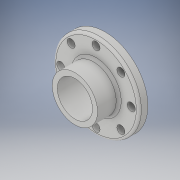
# Autodesk Inventor part: 410571040-T3
Saved by Autodesk Inventor 2017 (Build 210142000, 142)
## iProperties
Part Number: 410571040-T3
Material: 一般
Document SubType Name: Modeling
Designer: user
Density: 1 g/cm^3
Appearance: 預設
Author: user
Autodesk Inventor part; units mm, degrees
ref_plane "YZ Plane" through (0, 0, 0) normal (1, 0, 0) x (0, 1, 0)
ref_plane "XZ Plane" through (0, 0, 0) normal (0, 1, 0) x (-1, 0, 0)
ref_plane "XY Plane" through (0, 0, 0) normal (0, 0, 1) x (1, 0, 0)
sketch "草圖1" plane through (0, 0, 0) normal (1, 0, 0) x (0, 1, 0)
  line L0 (0, 0) -> (45, 0)
  line L1 (45, 0) -> (45, -42)
  line L2 (45, -42) -> (85, -42)
  line L3 (85, -42) -> (85, -60)
  line L4 (85, -60) -> (0, -60)
  line L5 (0, -60) -> (0, 0)
  dimension "d0" = 60
  dimension "d1" = 85
  dimension "d2" = 42
  dimension "d3" = 40
  constraints: 12 end point, 5 perpendicular, 1 horizontal
  measures "d0" distance of L4.end L0.start
  measures "d1" distance of L3.end L4.end
  measures "d2" distance of L0.end L1.end
  measures "d3" distance of L1.end L2.end
revolve "迴轉1" add sketch "草圖1" angle 360 about axis through (0, 0, -60) along (0, 0, 1)
sketch "草圖2" plane through (0, 0, -42) normal (0, 0, 1) x (1, 0, 0)
  circle A0 centre (0, 0) radius 70 construction
  circle A1 centre (0, 70) radius 8
  circle A2 centre (-49.4975, 49.4975) radius 8
  circle A3 centre (-70, 0) radius 8
  circle A4 centre (-49.4975, -49.4975) radius 8
  circle A5 centre (0, -70) radius 8
  circle A6 centre (49.4975, -49.4975) radius 8
  circle A7 centre (70, 0) radius 8
  circle A8 centre (49.4975, 49.4975) radius 8
  dimension "d5" = 140
  dimension "d6" = 16
  dimension "d7" = 70
  dimension "d12" = 360
  constraints: 8 centre point, 6 coincident, 1 vertical alignment, 25 other
  measures "d6" diameter of A1
  measures "d7" distance of A1.centre point (0, 0)
extrude "擠出1" cut sketch "草圖2" against normal up to next
sketch "草圖4" plane through (0, 0, 0) normal (0, 0, 1) x (1, 0, 0)
  circle A0 centre (0, 0) radius 35
  dimension "d14" = 70
  constraints: 1 centre point, 1 coincident
  measures "d14" diameter of A0
extrude "擠出2" cut sketch "草圖4" against normal up to next
fillet "圓角1" radius 5 2 edges at (0, -45, -42) (0, -85, -42)
